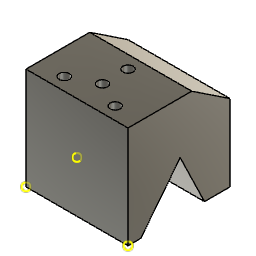
Suètone-drawing-object-03_02 v6 (Autodesk Fusion 360 design; units mm, degrees)
Autodesk Fusion 360 part; units mm, degrees
sketch "Esquisse1" plane through (0, 0, 0) normal (0, 0, 1) x (1, 0, 0)
  line L0 (40, 40) -> (-40, 40)
  line L1 (-40, 40) -> (-40, -40)
  line L2 (-40, -40) -> (40, -40)
  line L3 (40, -40) -> (40, 40)
  line L4 (40, 40) -> (-40, -40) construction
  line L5 (-40, 40) -> (40, -40) construction
  dimension "d1" = 80
  dimension "d2" = 80
  constraint horizontal L0
  constraint perpendicular L0 L1
  constraint parallel L0 L2
  constraint parallel L1 L3
  constraint coincident L4 origin
  constraint coincident L5 origin
  measures "d1" distance of L1.end L2.end
  measures "d2" distance of L0.end L1.end
extrude "Extrusion1" add sketch "Esquisse1" along normal blind 80 makes body 1
sketch "Esquisse4" plane through (0, 0, 80) normal (0, 0, 1) x (-1, 0, 0)
  line L0 (-40, 40) -> (-40, -40)
  line L1 (-40, -40) -> (40, -40)
  line L2 (40, -40) -> (40, 40)
  line L3 (40, 40) -> (-40, 40)
  circle A0 centre (0, 20) radius 4
  circle A1 centre (0, 0) radius 4
  circle A2 centre (-20, 30) radius 4
  circle A3 centre (20, 30) radius 4
  dimension "d5" = 8
  dimension "d6" = 8
  dimension "d7" = 8
  dimension "d8" = 8
  constraint coincident A1.centre origin
  measures "d5" diameter of A0
  measures "d6" diameter of A1
  measures "d7" diameter of A2
  measures "d8" diameter of A3
extrude "Extrusion2" cut sketch "Esquisse4" against normal blind 95 contours A0 | A1 | A2 | A3 bodies 1
sketch "Esquisse6" plane through (-40, 0, 20) normal (-1, 0, 0) x (0, -1, 0)
sketch "Esquisse8" plane through (40, 0, 0) normal (1, 0, 0) x (0, 1, 0)
  line L0 (-40, 0) -> (40, 0)
  line L1 (40, 0) -> (40, 80)
  line L2 (40, 80) -> (-40, 80)
  line L3 (-40, 80) -> (-40, 0)
  line L4 (-30, 0) -> (0.95, 39.3693)
  line L5 (40, 0) -> (20, 0)
  line L6 (0.95, 39.3693) -> (20, 0)
  dimension "d12" = 20
  constraint coincident L0.end L1.start
  constraint perpendicular L1 L5
  measures "d12" distance of L0.end L5.end
sketch "Esquisse9" plane through (0, -40, 0) normal (0, -1, 0) x (1, 0, 0)
  point P0 (40, 0)
  point P1 (0, 40)
  point P2 (-40, 0)
extrude "Extrusion3" cut sketch "Esquisse8" against normal blind 175 contours L0 L4 L6 bodies 1
sketch "Esquisse10" plane through (40, 0, 0) normal (1, 0, 0) x (0, 1, 0)
  line L0 (0.95, 39.3693) -> (20, 0)
  line L1 (20, 0) -> (40, 0)
  line L2 (40, 0) -> (40, 80)
  line L3 (40, 80) -> (-40, 80)
  line L4 (-40, 80) -> (-40, 0)
  line L5 (-40, 0) -> (-30, 0)
  line L6 (-30, 0) -> (0.95, 39.3693)
  line L7 (10, 80) -> (40, 60)
ref_plane "Plan de construction1" through (40, 25, 70) normal (0, -0.5547, -0.83205) x (0, 0.83205, -0.5547)
split "Scinder1" by plane through (40, 25, 70) normal (0, -0.5547, -0.83205) bodies 1 makes body 2 at (-13.3333, -40, 26.6667)
delete_body "RemoveBody1" bodies 1
